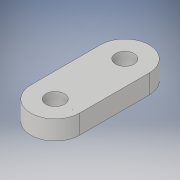
# Autodesk Inventor part: Rod_constraint
Saved by Autodesk Inventor 2019 (Build 230136000, 136)
## iProperties
Created: 2019-12-09
Part Number: Rod_constraint
Material: Generic
Document SubType Name: Modeling
Designer: Jorian Bruslind
Density: 1 g/cm^3
Appearance: Default
Author: Jorian Bruslind
Autodesk Inventor part; units mm, degrees
ref_plane "YZ Plane" through (0, 0, 0) normal (1, 0, 0) x (0, 1, 0)
ref_plane "XZ Plane" through (0, 0, 0) normal (0, 1, 0) x (-1, 0, 0)
ref_plane "XY Plane" through (0, 0, 0) normal (0, 0, 1) x (1, 0, 0)
sketch "Sketch1" plane through (0, 0, 0) normal (0, 1, 0) x (-1, 0, 0)
  line L0 (0, 0) -> (0, -20)
  line L1 (0, 0) -> (-4, 0) construction
  line L2 (0, -20) -> (-4, -20) construction
  line L3 (0, 0) -> (-5, 0)
  arc A0 (5, 0) -> (-5, 0) centre (0, 0) ccw
  line L4 (-5, 0) -> (-5, -20)
  arc A1 (-5, -20) -> (5, -20) centre (0, -20) ccw
  line L5 (5, -20) -> (5, 0)
  dimension "d11" = 20
  dimension "d12" = 5
  dimension "d13" = 90
  dimension "d14" = 20
  constraints: 12 end point, 4 coincident, 4 point on circle, 3 point on line, 3 vertical, 2 centre point
  measures "d11" distance of L1.start L2.start
  measures "d12" distance of L1.start L3.end
  measures "d13" angle of L1 L0
  measures "d14" distance of L3.end L4.end
sketch "Sketch1 outline for Extrusion1" plane through (0, 0, 0) normal (0, 1, 0) x (-1, 0, 0)
  arc A0 (-5, 0) -> (5, 0) centre (0, 0) cw
  line L0 (5, 0) -> (5, -20)
  arc A1 (5, -20) -> (-5, -20) centre (0, -20) cw
  line L1 (-5, -20) -> (-5, 0)
extrude "Extrusion1" add sketch "Sketch1 outline for Extrusion1" along normal blind 5.5
sketch "Sketch2" plane through (0, 5.5, 0) normal (0, 1, 0) x (1, 0, 0)
  circle A0 centre (0, 0) radius 2.655
  line L0 (0, 0) -> (0, 20)
  circle A1 centre (0, 20) radius 2.655
  dimension "d7" = 5.31
  dimension "d8" = 20
  dimension "d9" = 5.31
  constraints: 2 centre point, 2 coincident, 2 end point, 1 vertical
  measures "d7" diameter of A0
  measures "d8" distance of L0.start L0.end
  measures "d9" diameter of A1
sketch "Sketch3" plane through (0, 0, 0) normal (0, -1, 0) x (1, 0, 0)
  circle A0 centre (0, 0) radius 1.9
  line L0 (0, 0) -> (0, -20)
  circle A1 centre (0, -20) radius 1.9
  dimension "d15" = 3.8
  dimension "d16" = 20
  dimension "d17" = 3.8
  constraints: 2 centre point, 2 coincident, 2 end point, 1 vertical
  measures "d15" diameter of A0
  measures "d16" distance of L0.start L0.end
  measures "d17" diameter of A1
sketch "Sketch3 outline for Extrusion2" plane through (0, 0, 0) normal (0, -1, 0) x (1, 0, 0)
  circle A0 centre (0, 0) radius 1.9
  circle A1 centre (0, -20) radius 1.9
extrude "Extrusion2" cut sketch "Sketch3 outline for Extrusion2" against normal blind 1.2
sketch "Sketch4" plane through (0, 1.2, -20) normal (0, -1, 0) x (1, 0, 0)
  circle A0 centre (0, 0) radius 1.9 projected
  circle A1 centre (0, 0) radius 1.9
  circle A2 centre (0, 20) radius 1.9
  constraints: 2 centre point, 2 coincident
sketch "Sketch5" plane through (5, 0, 0) normal (1, 0, 0) x (0, 0, -1)
  line L0 (0, 0) -> (0, 5.5) projected
  line L1 (0, 0) -> (0, 5.5)
  constraints: 2 end point, 1 vertical
hole "Hole1" at (0, 5.5, 0) at (0, 5.5, -20) direction (0, -1, 0) diameter 5.1 depth 4 tip angle 118 countersink diameter 5.31 countersink angle 3.01
thicken "Thicken1" operation add thickness 2 both sides no extend neighbours yes toward (0.9967573, 0, -0.0804666) faces at (4.983787, 3.666667, -20.402333) (5, 1.833333, -13.333333) (-5, 1.833333, -6.666667) (-4.983787, 3.666667, 0.402333)
body "Solid1"
